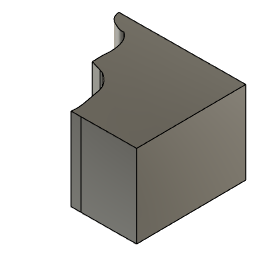
Version 9 (Autodesk Fusion 360 design; units mm, degrees)
Autodesk Fusion 360 part; units mm, degrees
note: some values were not read from the file. Set by a fixed rule: which sketch regions a step uses.
sketch "Sketch1" plane through (0, 0, 0) normal (0, 0, 1) x (1, 0, 0)
  line L0 (4.291, -19.3396) -> (5.2341, -19.3396)
  line L1 (20, 20) -> (19.9286, 19.9993)
  spline S0 degree 5 poles (-9.9419, 7.2762) (-9.9431, 7.2538) (-9.9572, 6.9879) (-9.9791, 6.5472) (-9.9981, 6.0998) (-10.0131, 5.6476) (-10.0208, 5.2183) (-10.0227, 5.0422) knots 0.054522 0.054522 0.054522 0.054522 0.054522 0.054522 0.057143 0.085714 0.105649 0.105649 0.105649 0.105649 0.105649 0.105649
  line L2 (-9.93, 7.4984) -> (-9.9538, 7.054)
  line L3 (-10.0202, 5.2727) -> (-10.0252, 4.8117)
  line L4 (-20.6927, 20.2862) -> (4.9343, 20.4792)
  spline S1 degree 5 poles (-20.6927, 20.2862) (-20.6865, 20.2134) (-20.6716, 20.0678) (-20.6416, 19.8492) (-20.586, 19.5574) (-20.4902, 19.1924) (-20.3668, 18.828) (-20.214, 18.4655) (-20.0287, 18.1076) (-19.8068, 17.758) (-19.5444, 17.4211) (-19.2389, 17.1012) (-18.8907, 16.8022) (-18.5041, 16.5269) (-18.0891, 16.276) (-17.6598, 16.0489) (-17.2317, 15.8441) (-16.819, 15.6599) (-16.4328, 15.4947) (-16.078, 15.3478) (-15.7513, 15.2198) (-15.4443, 15.1121) (-15.146, 15.0267) (-14.8452, 14.9651) (-14.5337, 14.9286) (-14.207, 14.9176) (-13.9316, 14.9293) (-13.7169, 14.9495) (-13.5701, 14.9681) (-13.4958, 14.9787) knots 0 0 0 0 0 0 0.04 0.08 0.12 0.16 0.2 0.24 0.28 0.32 0.36 0.4 0.44 0.48 0.52 0.56 0.6 0.64 0.68 0.72 0.76 0.8 0.84 0.88 0.92 0.96 1 1 1 1 1 1
  spline S2 degree 5 poles (-13.4958, 14.9787) (-13.4149, 14.9177) (-13.2402, 14.783) (-12.9744, 14.567) (-12.6252, 14.2568) (-12.2099, 13.8324) (-11.816, 13.3592) (-11.4605, 12.8507) (-11.1458, 12.3103) (-10.8722, 11.7424) (-10.6387, 11.1522) (-10.4433, 10.5455) (-10.283, 9.928) (-10.1552, 9.3051) (-10.0571, 8.6811) (-9.9869, 8.0593) (-9.9431, 7.4421) (-9.9247, 6.8309) (-9.931, 6.2266) (-9.9556, 5.7491) (-9.9849, 5.3943) (-10.0093, 5.1593) (-10.0227, 5.0422) knots 0.603172 0.603172 0.603172 0.603172 0.603172 0.603172 0.622222 0.644444 0.666667 0.688889 0.711111 0.733333 0.755556 0.777778 0.8 0.822222 0.844444 0.866667 0.888889 0.911111 0.933333 0.955556 0.977778 1 1 1 1 1 1
  line L5 (-14.4158, 15.6724) -> (-12.5759, 14.285)
  line L6 (-10.0227, 0.8939) -> (-10.0227, 0)
  line L7 (-10.0227, 0) -> (-4.8498, -1.5892)
  line L8 (4.7104, -19.3396) -> (3.0717, -19.3396)
  line L9 (3.0717, -19.3396) -> (2.0717, -19.3396)
  spline S3 degree 5 poles (-10.0227, 5.0422) (-10.0363, 4.8855) (-10.0599, 4.5653) (-10.0839, 4.0647) (-10.0959, 3.3602) (-10.0725, 2.4261) (-10.0442, 1.5406) (-10.0015, 0.9009) (-10.036, 0.6793) (-10.0409, 0.6139) (-10.0253, 0.5879) (-10.0227, 0.5844) knots 0 0 0 0 0 0 0.028571 0.057143 0.085714 0.114286 0.142857 0.171429 0.176045 0.176045 0.176045 0.176045 0.176045 0.176045
  line L10 (-10.0148, 1.2691) -> (-10.0307, 0.5187)
  line L11 (-10.1451, 0.7508) -> (-9.9004, 0.4181)
  line L12 (5.2341, -19.3396) -> (4.9343, 20.4792)
  line L13 (2.0717, -19.3396) -> (1.6192, -19.3396)
  spline S4 degree 5 poles (-6.626, -1.0435) (-6.5424, -1.0721) (-6.2954, -1.1535) (-5.9128, -1.2663) (-5.5695, -1.3544) (-5.2432, -1.4472) (-4.9811, -1.5385) (-4.8498, -1.5892) knots 0.300161 0.300161 0.300161 0.300161 0.300161 0.300161 0.314286 0.342857 0.371054 0.371054 0.371054 0.371054 0.371054 0.371054
  line L14 (-6.8411, -0.97) -> (-6.4109, -1.117)
  line L15 (-5.019, -1.5239) -> (-4.6805, -1.6545)
  spline S5 degree 5 poles (1.6192, -19.3396) (1.6522, -19.2025) (1.7116, -18.9219) (1.7808, -18.4815) (1.8332, -17.8553) (1.8331, -17.0083) (1.7699, -16.1002) (1.6497, -15.1378) (1.4827, -14.1328) (1.2853, -13.1037) (1.0765, -12.0728) (0.8736, -11.0628) (0.6886, -10.0934) (0.5237, -9.1778) (0.3678, -8.3197) (0.1914, -7.509) (-0.0443, -6.7281) (-0.3777, -5.9584) (-0.8362, -5.1873) (-1.4278, -4.414) (-2.1283, -3.6581) (-2.8895, -2.9538) (-3.6226, -2.3645) (-4.1665, -1.9858) (-4.5337, -1.7613) (-4.7548, -1.6391) (-4.8498, -1.5892) knots 0 0 0 0 0 0 0.033333 0.066667 0.1 0.133333 0.166667 0.2 0.233333 0.266667 0.3 0.333333 0.366667 0.4 0.433333 0.466667 0.5 0.533333 0.566667 0.6 0.633333 0.666667 0.7 0.726408 0.726408 0.726408 0.726408 0.726408 0.726408
  line L16 (-3.4988, -2.2989) -> (-6.2007, -0.8795)
  point P0 (-10.0227, 0.8939)
  point P1 (-12.1009, 13.6901)
  point P2 (-10.1967, 9.4856)
  point P3 (-20.2237, 18.5049)
  point P4 (-18.7992, 16.7452)
  point P5 (-16.4809, 15.5163)
  point P6 (-15, 15)
  point P7 (1.6192, -15)
  point P8 (0.5111, -9.1116)
  point P9 (-1, -5)
  constraint horizontal L0
  constraint midpoint S0.start L2
  constraint midpoint S0.end L3
  constraint midpoint S1.end L5
  constraint coincident P0 L6.start
  constraint vertical L6
  constraint coincident L7.end S4.end
  constraint coincident L0 L8.start
  constraint parallel L0 L8
  constraint coincident L6 S3.end
  constraint midpoint P0 L10
  constraint midpoint S3.end L11
  constraint coincident L7 S4.start
  constraint perpendicular L4 L12
  constraint parallel L9 L13
  constraint midpoint S4.start L14
  constraint midpoint L7.end L15
  constraint midpoint L7.end L16
extrude "Extrude1" add sketch "Sketch1" along normal blind 40 contours L0 L4 S1 S2 L6 L7 L8 L9 S3 L12 L13 S4 S5 picked at (-3.1113, 8.6204) makes body 1
delete_body "RemoveBody1" bodies 1
extrude "Extrude4" add sketch "Sketch1" along normal blind 30 separate body contours L0 L4 S1 S2 L6 L7 L8 L9 S3 L12 L13 S4 S5 picked at (-3.1113, 8.6204) makes body 2
extrude "Extrude5" add 1 faces at (5.1342, -6.0667, 10) along direction (0.999972, 0.007529, 0) blind 20 on bodies 2 bodies 2
